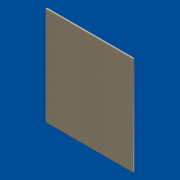
# Autodesk Inventor part: MDF_Base
Saved by Autodesk Inventor 2012 SP1 (Build 160190100, 190)
## iProperties
Created: 2012-05-08
Part Number: MDF_Base
Material: Default
Document SubType Name: Modeling
Designer: ERF
Density: 1 g/cm^3
Stock Number: SM-SWB
Description: MDF Waste Board
Project: Shapeoko
Vendor: various
Mass: 1143 g
Surface Area: 3707.95 cm^2
Volume: 1143 cm^3
Author: ERF
Title: 400mm x 450mm MDF
Autodesk Inventor part; units mm, degrees
ref_plane "YZ Plane" through (0, 0, 0) normal (1, 0, 0) x (0, 1, 0)
ref_plane "XZ Plane" through (0, 0, 0) normal (0, 1, 0) x (-1, 0, 0)
ref_plane "XY Plane" through (0, 0, 0) normal (0, 0, 1) x (1, 0, 0)
sketch "Sketch1" plane through (0, 0, 0) normal (0, 0, 1) x (1, 0, 0)
  line L0 (-200, 225) -> (200, 225)
  line L1 (200, 225) -> (200, -225)
  line L2 (200, -225) -> (-200, -225)
  line L3 (-200, -225) -> (-200, 225)
  point P0 (0, 0)
  dimension "d0" = 400
  dimension "d1" = 450
  dimension "d2" = 200
  dimension "d3" = 225
  constraints: 8 end point, 2 parallel, 1 horizontal, 1 perpendicular
  measures "d0" distance of L1.end L2.end
  measures "d1" distance of L0.end L1.end
  measures "d2" distance from line of L3 point (0, 0)
  measures "d3" distance from line of L0 point (0, 0)
extrude "Extrusion1" add sketch "Sketch1" along normal blind 6.35
body "Solid1"
